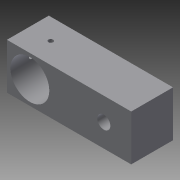
# Autodesk Inventor part: MotorBarConnect
Saved by Autodesk Inventor 2015 (Build 190159000, 159)
## iProperties
Created: 2016-05-04
Part Number: MotorBarConnect
Material: Generic
Document SubType Name: Modeling
Designer: Hatch
Density: 1 g/cm^3
Appearance: Default
Author: Hatch
Autodesk Inventor part; units mm, degrees
ref_plane "YZ Plane" through (0, 0, 0) normal (1, 0, 0) x (0, 1, 0)
ref_plane "XZ Plane" through (0, 0, 0) normal (0, 1, 0) x (-1, 0, 0)
ref_plane "XY Plane" through (0, 0, 0) normal (0, 0, 1) x (1, 0, 0)
sketch "Sketch1" plane through (0, 0, 0) normal (0, 1, 0) x (-1, 0, 0)
  circle A0 centre (0, 0) radius 14.875
  line L0 (-17.5, 17.5) -> (17.5, 17.5)
  line L1 (17.5, 17.5) -> (17.5, -17.5)
  line L2 (17.5, -17.5) -> (-17.5, -17.5)
  line L3 (-17.5, -17.5) -> (-17.5, 17.5)
  line L4 (-17.5, 17.5) -> (17.5, -17.5) construction
  line L5 (17.5, 17.5) -> (-17.5, -17.5) construction
  dimension "d0" = 29.75
  dimension "d1" = 35
  dimension "d2" = 35
  constraints: 12 end point, 2 midpoint, 2 parallel, 1 centre point, 1 coincident, 1 horizontal, 1 perpendicular
  measures "d0" diameter of A0
  measures "d1" distance of L1.end L2.end
  measures "d2" distance of L0.end L1.end
extrude "Extrusion1" add sketch "Sketch1" along normal blind 32
sketch "Sketch2" plane through (17.5, 0, 17.5) normal (1, 0, 0) x (0, 0, -1)
  line L0 (0, 0) -> (35, 0)
  line L1 (35, 0) -> (35, 32)
  line L2 (35, 32) -> (0, 32)
  line L3 (0, 32) -> (0, 0)
  point P0 (17.5, 0)
  constraints: 8 end point, 2 parallel, 1 horizontal, 1 perpendicular
sketch "Sketch3" plane through (0, 32, 0) normal (0, 1, 0) x (1, 0, 0)
  line L0 (17.5, -17.5) -> (17.5, 17.5) projected
  line L1 (17.5, 0) -> (56.57, 0)
  circle A0 centre (56.57, 0) radius 5
  point P0 (0, 0)
  dimension "d5" = 56.57
  dimension "d9" = 10
  constraints: 2 end point, 1 centre point, 1 coincident, 1 midpoint
  measures "d5" distance of point (0, 0) L1.end
  measures "d9" diameter of A0
extrude "Extrusion2" add sketch "Sketch2" along normal blind 60
extrude "Extrusion3" cut sketch "Sketch3" against normal through all
sketch "Sketch5" plane through (-17.5, 0, 17.5) normal (0, 0, 1) x (1, 0, 0)
  circle A0 centre (17.5, 16) radius 1.778
  point P0 (17.5, 0)
  dimension "d15" = 3.556
  constraints: 1 centre point
  measures "d15" diameter of A0
extrude "Extrusion5" cut sketch "Sketch5" against normal blind 10
sketch "Sketch6" plane through (-17.5, 0, -17.5) normal (-1, 0, 0) x (0, 0, 1)
  circle A0 centre (17.5, 16) radius 1.778
  point P0 (17.5, 0)
  dimension "d18" = 3.556
  constraints: 1 centre point
  measures "d18" diameter of A0
extrude "Extrusion6" cut sketch "Sketch6" against normal blind 3.556
equation "\"d19\" = d18"
body "Solid1"
